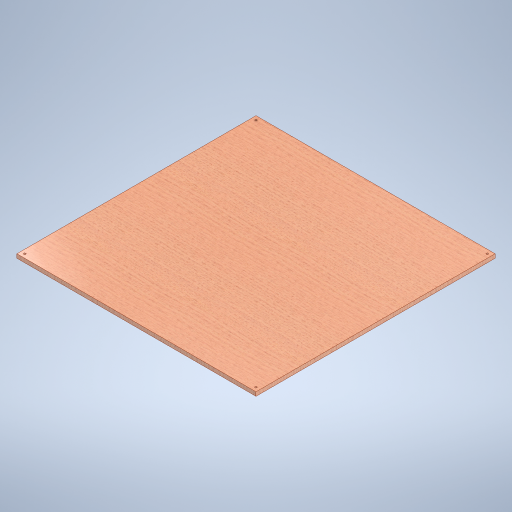
# Autodesk Inventor part: Soporte de matriz centelladora
Saved by Autodesk Inventor 2024.2 (Build 282272000, 272)
## iProperties
Created: 2024-08-22
Part Number: Soporte de matriz centelladora
Material: Wood (Oak)
Document SubType Name: Modeling
Designer: ja.restrepo1
Density: 0.76 g/cm^3
Appearance: White Oak - Natural Medium Gloss
Author: ja.restrepo1
Autodesk Inventor part; units mm, degrees
ref_plane "YZ Plane" through (0, 0, 0) normal (1, 0, 0) x (0, 1, 0)
ref_plane "XZ Plane" through (0, 0, 0) normal (0, 1, 0) x (-1, 0, 0)
ref_plane "XY Plane" through (0, 0, 0) normal (0, 0, 1) x (1, 0, 0)
sketch "Sketch1" plane through (0, 0, 0) normal (0, 1, 0) x (-1, 0, 0)
  line L0 (305, 305) -> (-305, 305)
  line L1 (-305, 305) -> (-305, -305)
  line L2 (-305, -305) -> (305, -305)
  line L3 (305, -305) -> (305, 305)
  circle A0 centre (295, 295) radius 2.5
  circle A1 centre (295, -295) radius 2.5
  circle A2 centre (-295, -295) radius 2.5
  circle A3 centre (-295, 295) radius 2.5
  line L4 (295, 295) -> (295, -295) construction
  line L5 (295, -295) -> (-295, -295) construction
  point P0 (0, 0)
  point P1 (305, 0)
  point P2 (0, 305)
  point P3 (295, 0)
  point P4 (0, -295)
  dimension "d0" = 610
  dimension "d1" = 5
  dimension "d2" = 590
  constraints: 12 end point, 4 centre point, 4 midpoint, 4 perpendicular, 3 equal radius, 3 horizontal alignment, 3 vertical alignment, 2 parallel, 1 horizontal, 1 vertical
  measures "d0" distance of L0.start L0.end
  measures "d1" diameter of A1
  measures "d2" distance of L4.end L5.end
extrude "Entrecentellas" add sketch "Sketch1" along normal mid plane 10
body "Solid1"
